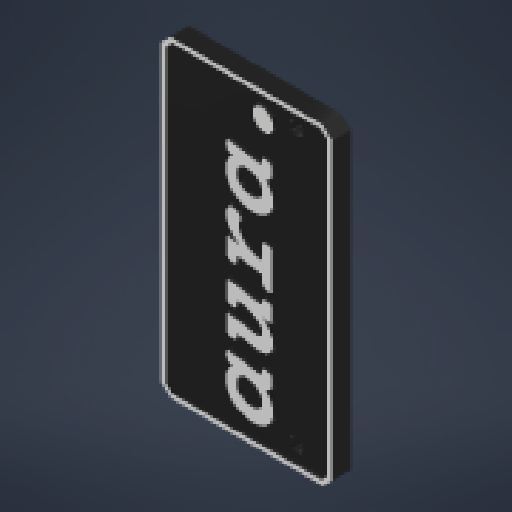
# Autodesk Inventor part: plate
Saved by Autodesk Inventor 2025.2 (Build 292293000, 293)
## iProperties
Created: 2025-11-18
Part Number: plate
Material: white pla
Document SubType Name: Modeling
Designer: cloudy
Density: 1 g/cm^3
Appearance: Smooth - Black
Author: cloudy
Autodesk Inventor part; units mm, degrees
ref_plane "YZ Plane" through (0, 0, 0) normal (1, 0, 0) x (0, 1, 0)
ref_plane "XZ Plane" through (0, 0, 0) normal (0, 1, 0) x (-1, 0, 0)
ref_plane "XY Plane" through (0, 0, 0) normal (0, 0, 1) x (1, 0, 0)
sketch "Sketch1" plane through (0, 0, 0) normal (0, 0, 1) x (1, 0, 0)
  circle A0 centre (12.7, -44.45) radius 2.1844 projected
  circle A1 centre (12.7, 44.45) radius 2.1844 projected
  circle A2 centre (-17.4625, 31.75) radius 2.1844 projected
  circle A3 centre (-17.4625, -31.75) radius 2.1844 projected
  line L0 (-30.1625, -50.8) -> (25.4, -50.8)
  line L1 (25.4, -50.8) -> (25.4, 50.8)
  line L2 (25.4, 50.8) -> (-30.1625, 50.8)
  line L3 (-30.1625, 50.8) -> (-30.1625, -50.8)
  line L4 (-29.3688, -50.8) -> (24.6062, -50.8) projected
  line L5 (-29.3688, 50.8) -> (24.6062, 50.8) projected
  line L6 (25.4, 51.5937) -> (25.4, 115.3993) projected
  line L7 (-30.1625, -171.45) -> (-30.1625, -51.5937) projected
  point P0 (0, 0)
  dimension "d9" = 101.6
  constraints: 8 end point, 3 collinear, 2 parallel, 1 horizontal, 1 perpendicular
  measures "d9" distance between parallel lines of L2 L0
extrude "Extrusion1" add sketch "Sketch1" along normal blind 5.08 contours A2 | A3 | L3 L2 L1 L0
sketch "Sketch2" plane through (0, 0, 5.08) normal (0, 0, 1) x (1, 0, 0)
  line L0 (-9.2726, -45.5724) -> (-9.2726, 85.8354) construction
  line L1 (-9.2726, 85.8354) -> (11.4441, 85.8354) construction
  line L2 (11.4441, 85.8354) -> (11.4441, -45.5724) construction
  line L3 (11.4441, -45.5724) -> (-9.2726, -45.5724) construction
  spline S0 degree 2 poles (3.8682, -32.9895) (5.1079, -34.1672) (6.2649, -36.8946) (6.2649, -38.2995) knots 0 0 0 1 2 2 2
  spline S1 degree 2 poles (6.2649, -38.2995) (6.2649, -39.7045) (5.2525, -41.9153) (3.5169, -43.4443) (1.1615, -44.2501) (-0.1815, -44.2501) knots 0 0 0 1 2 3 4 4 4
  spline S2 degree 2 poles (-0.1815, -44.2501) (-1.1939, -44.2501) (-3.3427, -43.7955) (-5.3469, -42.9071) (-7.1445, -41.5641) (-8.4875, -39.7252) (-9.2726, -37.4524) (-9.2726, -36.0474) knots 0 0 0 1 2 3 4 5 6 6 6
  spline S3 degree 2 poles (-9.2726, -36.0474) (-9.2726, -34.4978) (-7.8263, -32.1011) (-6.5659, -31.5019) knots 0 0 0 1 2 2 2
  line L4 (-6.5659, -31.5019) -> (-8.0742, -31.2333)
  spline S4 degree 2 poles (-8.0742, -31.2333) (-8.6114, -31.1506) (-9.0866, -30.1795) (-9.0866, -29.2704) knots 0 0 0 1 2 2 2
  spline S5 degree 2 poles (-9.0866, -29.2704) (-9.0866, -28.3613) (-8.6114, -27.7828) (-8.0742, -27.8654) knots 0 0 0 1 2 2 2
  line L5 (-8.0742, -27.8654) -> (1.2648, -29.4977)
  spline S6 degree 2 poles (1.2648, -29.4977) (1.9053, -29.6423) (2.6285, -29.2084) (2.6285, -28.6919) knots 0 0 0 1 2 2 2
  line L6 (2.6285, -28.6919) -> (2.6285, -28.2167)
  spline S7 degree 2 poles (2.6285, -28.2167) (2.6285, -27.9481) (2.7525, -27.5968) (3.1244, -27.4109) (3.7649, -27.4109) (4.2814, -27.5142) knots 0 0 0 1 2 3 4 4 4
  spline S8 degree 2 poles (4.2814, -27.5142) (4.798, -27.6175) (5.4385, -27.8241) (5.7897, -28.134) (5.9137, -28.5266) (5.9137, -28.7952) knots 0 0 0 1 2 3 4 4 4
  line L7 (5.9137, -28.7952) -> (5.9137, -30.3242)
  spline S9 degree 2 poles (5.9137, -30.3242) (5.9137, -30.7994) (5.7071, -31.6878) (5.2319, -32.3903) (4.4467, -32.8862) (3.8682, -32.9895) knots 0 0 0 1 2 3 4 4 4
  spline S10 degree 2 poles (2.6285, -37.3285) (2.6285, -36.254) (1.6987, -34.5805) (0.2317, -33.4234) (-1.5865, -32.8242) (-2.4749, -32.8242) knots 0 0 0 1 2 3 4 4 4
  spline S11 degree 2 poles (-2.4749, -32.8242) (-3.2394, -32.8242) (-4.4378, -33.2788) (-5.2229, -34.1052) (-5.6362, -35.221) (-5.6362, -35.8821) knots 0 0 0 1 2 3 4 4 4
  spline S12 degree 2 poles (-5.6362, -35.8821) (-5.6362, -36.9772) (-4.5824, -38.5268) (-2.9915, -39.5186) (-1.1319, -39.9731) (-0.3674, -39.9731) knots 0 0 0 1 2 3 4 4 4
  spline S13 degree 2 poles (-0.3674, -39.9731) (1.0375, -39.9731) (2.6285, -38.5888) (2.6285, -37.3285) knots 0 0 0 1 2 2 2
  spline S14 degree 2 poles (2.5665, -13.2164) (4.5294, -14.642) (6.2649, -17.4933) (6.2649, -19.0016) knots 0 0 0 1 2 2 2
  spline S15 degree 2 poles (6.2649, -19.0016) (6.2649, -19.9727) (5.6244, -21.5017) (4.488, -22.5554) (2.8764, -23.1339) (1.9053, -23.1339) knots 0 0 0 1 2 3 4 4 4
  spline S16 degree 2 poles (1.9053, -23.1339) (1.6161, -23.1339) (1.0375, -23.0926) (0.707, -23.0306) knots 0 0 0 1 2 2 2
  line L8 (0.707, -23.0306) -> (-5.6362, -21.9149)
  line L9 (-5.6362, -21.9149) -> (-5.6362, -23.1546)
  spline S17 degree 2 poles (-5.6362, -23.1546) (-5.6362, -23.4232) (-5.7601, -23.7744) (-6.132, -23.9604) (-6.7725, -23.9604) (-7.2891, -23.8777) knots 0 0 0 1 2 3 4 4 4
  spline S18 degree 2 poles (-7.2891, -23.8777) (-7.8056, -23.7744) (-8.4461, -23.5472) (-8.7974, -23.2372) (-8.9213, -22.8447) (-8.9213, -22.5761) knots 0 0 0 1 2 3 4 4 4
  line L10 (-8.9213, -22.5761) -> (-8.9213, -18.3404)
  spline S19 degree 2 poles (-8.9213, -18.3404) (-8.9213, -17.8032) (-8.4461, -17.4107) (-7.9089, -17.514) knots 0 0 0 1 2 2 2
  line L11 (-7.9089, -17.514) -> (0.0871, -18.8983)
  spline S20 degree 2 poles (0.0871, -18.8983) (0.6037, -19.0016) (1.0169, -19.0016) knots 0 0 0 1 1 1
  spline S21 degree 2 poles (1.0169, -19.0016) (1.802, -19.0016) (2.6285, -18.3198) (2.6285, -17.4726) knots 0 0 0 1 2 2 2
  spline S22 degree 2 poles (2.6285, -17.4726) (2.6285, -16.7495) (1.5747, -15.2412) (-0.1608, -13.9395) (-2.351, -12.9684) (-3.508, -12.7825) knots 0 0 0 1 2 3 4 4 4
  line L12 (-3.508, -12.7825) -> (-5.6362, -12.4106)
  line L13 (-5.6362, -12.4106) -> (-5.6362, -14.1461)
  spline S23 degree 2 poles (-5.6362, -14.1461) (-5.6362, -14.4147) (-5.7601, -14.766) (-6.132, -14.9519) (-6.7725, -14.9519) (-7.2891, -14.8693) knots 0 0 0 1 2 3 4 4 4
  spline S24 degree 2 poles (-7.2891, -14.8693) (-7.8056, -14.766) (-8.4461, -14.5387) (-8.7974, -14.2288) (-8.9213, -13.8362) (-8.9213, -13.5676) knots 0 0 0 1 2 3 4 4 4
  line L14 (-8.9213, -13.5676) -> (-8.9213, -8.8361)
  spline S25 degree 2 poles (-8.9213, -8.8361) (-8.9213, -8.2989) (-8.4461, -7.9063) (-7.9089, -8.0096) knots 0 0 0 1 2 2 2
  line L15 (-7.9089, -8.0096) -> (2.6285, -9.8485)
  line L16 (2.6285, -9.8485) -> (2.6285, -8.6088)
  spline S26 degree 2 poles (2.6285, -8.6088) (2.6285, -8.3402) (2.7525, -7.989) (3.1037, -7.803) (3.7442, -7.803) (4.2608, -7.8857) knots 0 0 0 1 2 3 4 4 4
  spline S27 degree 2 poles (4.2608, -7.8857) (4.7773, -7.989) (5.4178, -8.2162) (5.7897, -8.5262) (5.9137, -8.9187) (5.9137, -9.1873) knots 0 0 0 1 2 3 4 4 4
  line L17 (5.9137, -9.1873) -> (5.9137, -12.7825)
  spline S28 degree 2 poles (5.9137, -12.7825) (5.9137, -13.3403) (5.4385, -13.7122) (4.9013, -13.6296) knots 0 0 0 1 2 2 2
  line L18 (4.9013, -13.6296) -> (2.5665, -13.2164)
  spline S29 degree 2 poles (-8.9213, 3.2509) (-8.9213, 3.8088) (-8.4461, 4.1807) (-7.9089, 4.0981) knots 0 0 0 1 2 2 2
  line L19 (-7.9089, 4.0981) -> (-4.5824, 3.5195)
  spline S30 degree 2 poles (-4.5824, 3.5195) (-6.9172, 5.1105) (-9.2726, 8.499) (-9.2726, 10.0693) knots 0 0 0 1 2 2 2
  spline S31 degree 2 poles (-9.2726, 10.0693) (-9.2726, 11.3916) (-8.3635, 12.5073) knots 0 0 0 1 1 1
  spline S32 degree 2 poles (-8.3635, 12.5073) (-7.9296, 13.0859) (-6.6899, 13.1685) (-5.7808, 12.652) knots 0 0 0 1 2 2 2
  spline S33 degree 2 poles (-5.7808, 12.652) (-4.8097, 12.1148) (-4.1898, 11.0817) (-4.4584, 10.6271) knots 0 0 0 1 2 2 2
  spline S34 degree 2 poles (-4.4584, 10.6271) (-4.913, 9.842) (-4.913, 8.9122) knots 0 0 0 1 1 1
  spline S35 degree 2 poles (-4.913, 8.9122) (-4.913, 7.9618) (-3.9832, 6.0403) (-2.3303, 4.3873) (-0.0575, 3.1683) (1.2648, 2.941) knots 0 0 0 1 2 3 4 4 4
  line L20 (1.2648, 2.941) -> (2.6285, 2.7344)
  line L21 (2.6285, 2.7344) -> (2.6285, 7.3419)
  spline S36 degree 2 poles (2.6285, 7.3419) (2.6285, 7.6105) (2.7525, 7.9618) (3.1244, 8.1271) (3.7649, 8.1271) (4.2814, 8.0444) knots 0 0 0 1 2 3 4 4 4
  spline S37 degree 2 poles (4.2814, 8.0444) (4.798, 7.9411) (5.4385, 7.7345) (5.7897, 7.4246) (5.9137, 7.032) (5.9137, 6.7634) knots 0 0 0 1 2 3 4 4 4
  line L22 (5.9137, 6.7634) -> (5.9137, -4.2286)
  spline S38 degree 2 poles (5.9137, -4.2286) (5.9137, -4.4972) (5.7897, -4.8691) (5.4385, -5.0344) (4.798, -5.055) (4.2814, -4.9724) knots 0 0 0 1 2 3 4 4 4
  spline S39 degree 2 poles (4.2814, -4.9724) (3.7649, -4.8691) (3.1244, -4.6418) (2.7525, -4.3319) (2.6285, -3.9186) (2.6285, -3.65) knots 0 0 0 1 2 3 4 4 4
  line L23 (2.6285, -3.65) -> (2.6285, -1.2946)
  line L24 (2.6285, -1.2946) -> (-5.6362, 0.1517)
  line L25 (-5.6362, 0.1517) -> (-5.6362, -1.7285)
  spline S40 degree 2 poles (-5.6362, -1.7285) (-5.6362, -1.9971) (-5.7601, -2.3484) (-6.1114, -2.5343) (-6.7519, -2.5343) (-7.2684, -2.4517) knots 0 0 0 1 2 3 4 4 4
  spline S41 degree 2 poles (-7.2684, -2.4517) (-7.785, -2.3484) (-8.4255, -2.1211) (-8.7974, -1.8112) (-8.9213, -1.4186) (-8.9213, -1.15) knots 0 0 0 1 2 3 4 4 4
  line L26 (-8.9213, -1.15) -> (-8.9213, 3.2509)
  spline S42 degree 2 poles (3.8682, 26.144) (5.1079, 24.9663) (6.2649, 22.239) (6.2649, 20.834) knots 0 0 0 1 2 2 2
  spline S43 degree 2 poles (6.2649, 20.834) (6.2649, 19.429) (5.2525, 17.2182) (3.5169, 15.6892) (1.1615, 14.8834) (-0.1815, 14.8834) knots 0 0 0 1 2 3 4 4 4
  spline S44 degree 2 poles (-0.1815, 14.8834) (-1.1939, 14.8834) (-3.3427, 15.338) (-5.3469, 16.2264) (-7.1445, 17.5694) (-8.4875, 19.4083) (-9.2726, 21.6811) (-9.2726, 23.0861) knots 0 0 0 1 2 3 4 5 6 6 6
  spline S45 degree 2 poles (-9.2726, 23.0861) (-9.2726, 24.6357) (-7.8263, 27.0324) (-6.5659, 27.6316) knots 0 0 0 1 2 2 2
  line L27 (-6.5659, 27.6316) -> (-8.0742, 27.9002)
  spline S46 degree 2 poles (-8.0742, 27.9002) (-8.6114, 27.9829) (-9.0866, 28.954) (-9.0866, 29.8631) knots 0 0 0 1 2 2 2
  spline S47 degree 2 poles (-9.0866, 29.8631) (-9.0866, 30.7722) (-8.6114, 31.3507) (-8.0742, 31.2681) knots 0 0 0 1 2 2 2
  line L28 (-8.0742, 31.2681) -> (1.2648, 29.6358)
  spline S48 degree 2 poles (1.2648, 29.6358) (1.9053, 29.4912) (2.6285, 29.9251) (2.6285, 30.4416) knots 0 0 0 1 2 2 2
  line L29 (2.6285, 30.4416) -> (2.6285, 30.9168)
  spline S49 degree 2 poles (2.6285, 30.9168) (2.6285, 31.1854) (2.7525, 31.5367) (3.1244, 31.7226) (3.7649, 31.7226) (4.2814, 31.6193) knots 0 0 0 1 2 3 4 4 4
  spline S50 degree 2 poles (4.2814, 31.6193) (4.798, 31.516) (5.4385, 31.3094) (5.7897, 30.9995) (5.9137, 30.6069) (5.9137, 30.3383) knots 0 0 0 1 2 3 4 4 4
  line L30 (5.9137, 30.3383) -> (5.9137, 28.8093)
  spline S51 degree 2 poles (5.9137, 28.8093) (5.9137, 28.3341) (5.7071, 27.4457) (5.2319, 26.7432) (4.4467, 26.2473) (3.8682, 26.144) knots 0 0 0 1 2 3 4 4 4
  spline S52 degree 2 poles (2.6285, 21.8051) (2.6285, 22.8795) (1.6987, 24.5531) (0.2317, 25.7101) (-1.5865, 26.3093) (-2.4749, 26.3093) knots 0 0 0 1 2 3 4 4 4
  spline S53 degree 2 poles (-2.4749, 26.3093) (-3.2394, 26.3093) (-4.4378, 25.8547) (-5.2229, 25.0283) (-5.6362, 23.9125) (-5.6362, 23.2514) knots 0 0 0 1 2 3 4 4 4
  spline S54 degree 2 poles (-5.6362, 23.2514) (-5.6362, 22.1563) (-4.5824, 20.6067) (-2.9915, 19.6149) (-1.1319, 19.1604) (-0.3674, 19.1604) knots 0 0 0 1 2 3 4 4 4
  spline S55 degree 2 poles (-0.3674, 19.1604) (1.0375, 19.1604) (2.6285, 20.5447) (2.6285, 21.8051) knots 0 0 0 1 2 2 2
  spline S56 degree 2 poles (6.2649, 42.0948) (6.2649, 41.4542) (5.7897, 40.3798) (5.0046, 39.5947) (3.9302, 39.1608) (3.331, 39.1608) knots 0 0 0 1 2 3 4 4 4
  spline S57 degree 2 poles (3.331, 39.1608) (2.5252, 39.1608) (1.1615, 39.7807) (0.1491, 40.8551) (-0.4088, 42.2187) (-0.4088, 42.9625) knots 0 0 0 1 2 3 4 4 4
  spline S58 degree 2 poles (-0.4088, 42.9625) (-0.4088, 43.6031) (0.0665, 44.6775) (0.8516, 45.4419) (1.926, 45.8758) (2.5045, 45.8758) knots 0 0 0 1 2 3 4 4 4
  spline S59 degree 2 poles (2.5045, 45.8758) (3.3103, 45.8758) (4.674, 45.256) (5.6864, 44.2229) (6.2649, 42.8386) (6.2649, 42.0948) knots 0 0 0 1 2 3 4 4 4
  point P0 (0, 0)
  constraints: 2 other
chamfer "Chamfer1" distance 3 angle 45 4 edges at (-30.1625, -50.8, 2.54) (-30.1625, 50.8, 2.54) (25.4, 50.8, 2.54) (25.4, -50.8, 2.54)
emboss "Emboss1" sketch "Sketch2" operation add depth 1 direction (0, 0, -1)
sketch "Sketch3" plane through (0, 0, 5.08) normal (0, 0, 1) x (1, 0, 0)
  circle A0 centre (12.7, 44.45) radius 2.1844 projected
  circle A1 centre (12.7, -44.45) radius 2.1844 projected
  line L0 (25.4, -47.8) -> (22.4, -50.8) projected
  line L1 (25.4, -47.8) -> (25.4, 47.8) projected
  line L2 (22.4, 50.8) -> (25.4, 47.8) projected
  line L3 (22.4, 50.8) -> (-27.1625, 50.8) projected
  line L4 (-30.1625, 47.8) -> (-27.1625, 50.8) projected
  line L5 (-30.1625, 47.8) -> (-30.1625, -47.8) projected
  line L6 (-27.1625, -50.8) -> (-30.1625, -47.8) projected
  line L7 (-27.1625, -50.8) -> (22.4, -50.8) projected
  line L8 (5.9137, 6.7634) -> (5.9137, -4.2286) projected
  line L9 (2.6285, -3.65) -> (2.6285, -1.2946) projected
  line L10 (2.6285, -1.2946) -> (-5.6362, 0.1517) projected
  line L11 (-5.6362, 0.1517) -> (-5.6362, -1.7285) projected
  line L12 (-8.9213, -1.15) -> (-8.9213, 3.2509) projected
  line L13 (-7.9089, 4.0981) -> (-4.5824, 3.5195) projected
  line L14 (1.2648, 2.941) -> (2.6285, 2.7344) projected
  line L15 (2.6285, 2.7344) -> (2.6285, 7.3419) projected
  line L16 (2.6285, 30.4416) -> (2.6285, 30.9168) projected
  line L17 (5.9137, 30.3383) -> (5.9137, 28.8093) projected
  line L18 (-6.5659, 27.6316) -> (-8.0742, 27.9002) projected
  line L19 (-8.0742, 31.2681) -> (1.2648, 29.6358) projected
  line L20 (2.6285, -28.6919) -> (2.6285, -28.2167) projected
  line L21 (5.9137, -28.7952) -> (5.9137, -30.3242) projected
  line L22 (-6.5659, -31.5019) -> (-8.0742, -31.2333) projected
  line L23 (-8.0742, -27.8654) -> (1.2648, -29.4977) projected
  line L24 (-8.9213, -13.5676) -> (-8.9213, -8.8361) projected
  line L25 (-7.9089, -8.0096) -> (2.6285, -9.8485) projected
  line L26 (2.6285, -9.8485) -> (2.6285, -8.6088) projected
  line L27 (5.9137, -9.1873) -> (5.9137, -12.7825) projected
  line L28 (4.9013, -13.6296) -> (2.5665, -13.2164) projected
  line L29 (0.707, -23.0306) -> (-5.6362, -21.9149) projected
  line L30 (-5.6362, -21.9149) -> (-5.6362, -23.1546) projected
  line L31 (-8.9213, -22.5761) -> (-8.9213, -18.3404) projected
  line L32 (-7.9089, -17.514) -> (0.0871, -18.8983) projected
  line L33 (-3.508, -12.7825) -> (-5.6362, -12.4106) projected
  line L34 (-5.6362, -12.4106) -> (-5.6362, -14.1461) projected
  line L35 (23.9, -47.3) -> (23.9, 47.3)
  line L36 (21.9, 49.3) -> (-26.6625, 49.3)
  line L37 (-28.6625, 47.3) -> (-28.6625, -47.3)
  line L38 (-26.6625, -49.3) -> (21.9, -49.3)
  line L39 (-26.6625, 49.3) -> (-28.6625, 47.3)
  line L40 (21.9, 49.3) -> (23.9, 47.3)
  line L41 (23.9, -47.3) -> (21.9, -49.3)
  line L42 (-26.6625, -49.3) -> (-28.6625, -47.3)
  point P0 (0, 0)
  point P1 (23.9, -49.3)
  point P2 (23.9, 49.3)
  point P3 (-28.6625, 49.3)
  point P4 (-28.6625, -49.3)
  dimension "d10" = 1.5
  dimension "d11" = 2
  dimension "d12" = 2
  dimension "d13" = 2
  dimension "d14" = 2
  dimension "d15" = 2
  dimension "d16" = 2
  dimension "d17" = 2
  dimension "d18" = 2
  constraints: 16 end point, 8 point on line, 55 other
  measures "d10" distance between parallel lines of L7 L38
  measures "d11" distance of L36.end point (-28.663, 49.3)
  measures "d12" distance of L37.start point (-28.663, 49.3)
  measures "d13" distance of L36.start point (23.9, 49.3)
  measures "d14" distance of L35.end point (23.9, 49.3)
  measures "d15" distance of L35.start point (23.9, -49.3)
  measures "d16" distance of L38.end point (23.9, -49.3)
  measures "d17" distance of L38.start point (-28.663, -49.3)
  measures "d18" distance of L37.end point (-28.663, -49.3)
extrude "Extrusion2" add sketch "Sketch3" along normal blind 1 contours L0 L7 L6 L5 L4 L3 L2 L1
equation "\"d12\" = d11"
equation "\"d13\" = d11"
equation "\"d14\" = d13"
equation "\"d15\" = d11"
equation "\"d16\" = d15"
equation "\"d17\" = d11"
equation "\"d18\" = d17"
body "Solid1"
